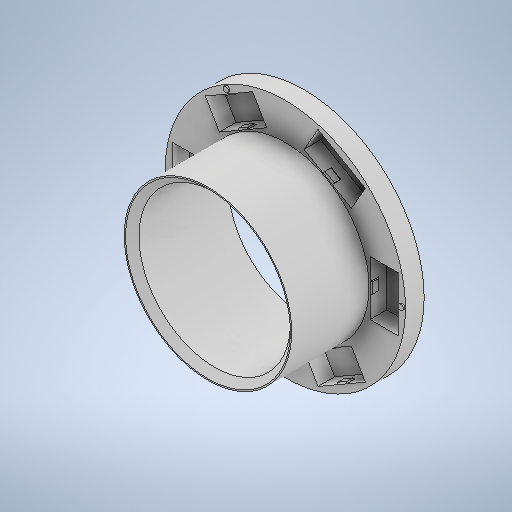
# Autodesk Inventor part: 2.5inchFemale
Saved by Autodesk Inventor 2025.2 (Build 292293000, 293)
## iProperties
Created: 2024-12-23
Part Number: 2.5inchFemale
Material: Generic
Document SubType Name: Modeling
Designer: lidang
Density: 1 g/cm^3
Appearance: Default
Author: lidang
Autodesk Inventor part; units mm, degrees
ref_plane "YZ Plane" through (0, 0, 0) normal (1, 0, 0) x (0, 1, 0)
ref_plane "XZ Plane" through (0, 0, 0) normal (0, 1, 0) x (-1, 0, 0)
ref_plane "XY Plane" through (0, 0, 0) normal (0, 0, 1) x (1, 0, 0)
sketch "Sketch1" plane through (0, 0, 0) normal (0, 0, 1) x (1, 0, 0)
  circle A0 centre (0, 0) radius 28.35
  line L0 (31.75, 10.25) -> (42.25, 10.25)
  line L1 (42.25, 10.25) -> (42.25, -10.25)
  line L2 (42.25, -10.25) -> (31.75, -10.25)
  line L3 (31.75, -10.25) -> (31.75, 10.25)
  circle A1 centre (0, 0) radius 45
  line L4 (42.25, 2) -> (41.75, 2)
  line L5 (41.75, 2) -> (41.75, -2)
  line L6 (41.75, -2) -> (42.25, -2)
  line L7 (42.25, -2) -> (42.25, 2)
  line L8 (37, 10.25) -> (37, -10.25)
  line L9 (31.75, 2) -> (32.25, 2)
  line L10 (32.25, 2) -> (32.25, -2)
  line L11 (32.25, -2) -> (31.75, -2)
  line L12 (31.75, -2) -> (31.75, 2)
  line L13 (19.3929, 37.5896) -> (19.1429, 37.1566)
  line L14 (22.6071, 35.1566) -> (22.8571, 35.5896)
  line L15 (22.8571, 35.5896) -> (19.3929, 37.5896)
  line L16 (19.1429, 37.1566) -> (22.6071, 35.1566)
  line L17 (14.1429, 28.4963) -> (14.3929, 28.9293)
  line L18 (14.3929, 28.9293) -> (17.8571, 26.9293)
  line L19 (17.6071, 26.4963) -> (14.1429, 28.4963)
  line L20 (17.8571, 26.9293) -> (17.6071, 26.4963)
  line L21 (24.7518, 22.3713) -> (6.9982, 32.6213)
  line L22 (30.0018, 31.4646) -> (24.7518, 22.3713)
  line L23 (12.2482, 41.7146) -> (30.0018, 31.4646)
  line L24 (6.9982, 32.6213) -> (12.2482, 41.7146)
  line L25 (-22.8571, 35.5896) -> (-22.6071, 35.1566)
  line L26 (-19.1429, 37.1566) -> (-19.3929, 37.5896)
  line L27 (-19.3929, 37.5896) -> (-22.8571, 35.5896)
  line L28 (-22.6071, 35.1566) -> (-19.1429, 37.1566)
  line L29 (-17.6071, 26.4963) -> (-17.8571, 26.9293)
  line L30 (-17.8571, 26.9293) -> (-14.3929, 28.9293)
  line L31 (-14.1429, 28.4963) -> (-17.6071, 26.4963)
  line L32 (-14.3929, 28.9293) -> (-14.1429, 28.4963)
  line L33 (-6.9982, 32.6213) -> (-24.7518, 22.3713)
  line L34 (-12.2482, 41.7146) -> (-6.9982, 32.6213)
  line L35 (-30.0018, 31.4646) -> (-12.2482, 41.7146)
  line L36 (-24.7518, 22.3713) -> (-30.0018, 31.4646)
  line L37 (-42.25, -2) -> (-41.75, -2)
  line L38 (-41.75, 2) -> (-42.25, 2)
  line L39 (-42.25, 2) -> (-42.25, -2)
  line L40 (-41.75, -2) -> (-41.75, 2)
  line L41 (-31.75, -2) -> (-32.25, -2)
  line L42 (-32.25, -2) -> (-32.25, 2)
  line L43 (-31.75, 2) -> (-31.75, -2)
  line L44 (-32.25, 2) -> (-31.75, 2)
  line L45 (-31.75, 10.25) -> (-31.75, -10.25)
  line L46 (-42.25, 10.25) -> (-31.75, 10.25)
  line L47 (-42.25, -10.25) -> (-42.25, 10.25)
  line L48 (-31.75, -10.25) -> (-42.25, -10.25)
  line L49 (-19.3929, -37.5896) -> (-19.1429, -37.1566)
  line L50 (-22.6071, -35.1566) -> (-22.8571, -35.5896)
  line L51 (-22.8571, -35.5896) -> (-19.3929, -37.5896)
  line L52 (-19.1429, -37.1566) -> (-22.6071, -35.1566)
  line L53 (-14.1429, -28.4963) -> (-14.3929, -28.9293)
  line L54 (-14.3929, -28.9293) -> (-17.8571, -26.9293)
  line L55 (-17.6071, -26.4963) -> (-14.1429, -28.4963)
  line L56 (-17.8571, -26.9293) -> (-17.6071, -26.4963)
  line L57 (-24.7518, -22.3713) -> (-6.9982, -32.6213)
  line L58 (-30.0018, -31.4646) -> (-24.7518, -22.3713)
  line L59 (-12.2482, -41.7146) -> (-30.0018, -31.4646)
  line L60 (-6.9982, -32.6213) -> (-12.2482, -41.7146)
  line L61 (22.8571, -35.5896) -> (22.6071, -35.1566)
  line L62 (19.1429, -37.1566) -> (19.3929, -37.5896)
  line L63 (19.3929, -37.5896) -> (22.8571, -35.5896)
  line L64 (22.6071, -35.1566) -> (19.1429, -37.1566)
  line L65 (17.6071, -26.4963) -> (17.8571, -26.9293)
  line L66 (17.8571, -26.9293) -> (14.3929, -28.9293)
  line L67 (14.1429, -28.4963) -> (17.6071, -26.4963)
  line L68 (14.3929, -28.9293) -> (14.1429, -28.4963)
  line L69 (6.9982, -32.6213) -> (24.7518, -22.3713)
  line L70 (12.2482, -41.7146) -> (6.9982, -32.6213)
  line L71 (30.0018, -31.4646) -> (12.2482, -41.7146)
  line L72 (24.7518, -22.3713) -> (30.0018, -31.4646)
  circle A2 centre (0, 0) radius 31.35
  point P0 (27.3768, 26.9179)
  point P1 (9.6232, 37.1679)
  point P2 (-9.6232, 37.1679)
  point P3 (-27.3768, 26.9179)
  point P4 (-37, 10.25)
  point P5 (-37, -10.25)
  point P6 (-27.3768, -26.9179)
  point P7 (-9.6232, -37.1679)
  point P8 (9.6232, -37.1679)
  point P9 (27.3768, -26.9179)
  dimension "d1" = 56.7
  dimension "d16" = 20.5
  dimension "d17" = 10.5
  dimension "d72" = 10.25
  dimension "d73" = 90
  dimension "d74" = 4
  dimension "d75" = 0.5
  dimension "d76" = 2
  dimension "d83" = 360
  dimension "d85" = 62.7
  dimension "d114" = 37
  constraints: 146 end point, 6 point on line, 4 parallel, 4 symmetric about line, 3 centre point, 2 horizontal, 2 midpoint, 2 perpendicular, 1 coincident, 157 other
  measures "d1" diameter of A0
  measures "d16" distance of L0.end L1.end
  measures "d17" distance of L1.end L2.end
  measures "d72" vertical distance of point (0, 0) L8.start
  measures "d73" diameter of A1
  measures "d74" distance of L4.end L5.end
  measures "d75" distance of L5.end L6.end
  measures "d76" vertical distance of point (0, 0) L5.end
  measures "d85" diameter of A2
  measures "d114" horizontal distance of point (0, 0) L8.start
extrude "Extrusion9" add sketch "Sketch1" along normal blind 7 contours A0 | L0 L8 L2 L3 L11 L10 L9 | L0 L1 L4 L5 L6 L2 L8 | L9 L10 L11 L3 | L1 L6 L5 L4 | A1 | L15 L14 L16 L13 | L13 L16 L14 L23 L22 L21 L20 L18 L17 L24 | L17 L18 L20 L19 | L27 L26 L28 L25 | L25 L28 L26 L35 L34 L33 L32 L30 L29 L36 | L29 L30 L32 L31 | L39 L38 L40 L37 | L37 L40 L38 L47 L46 L45 L44 L42 L41 L48 | L41 L42 L44 L43 | L51 L50 L52 L49 | L49 L52 L50 L59 L58 L57 L56 L54 L53 L60 | L53 L54 L56 L55 | L63 L62 L64 L61 | L61 L64 L62 L71 L70 L69 L68 L66 L65 L72 | L65 L66 L68 L67 | A2
extrude "Extrusion10" add sketch "Sketch1" along normal blind 36 contours A0 | A2
extrude "Extrusion11" cut sketch "Sketch1" along normal blind 36 contours A0
extrude "Extrusion12" cut sketch "Sketch1" along normal blind 7 contours L39 L38 L40 L37 | L37 L40 L38 L47 L46 L45 L44 L42 L41 L48 | L41 L42 L44 L43
extrude "Extrusion13" add sketch "Sketch1" along normal blind 7 contours L39 L38 L40 L37 | L41 L42 L44 L43
extrude "Extrusion14" add sketch "Sketch1" along normal blind 0.75 contours L39 L38 L40 L37 | L37 L40 L38 L47 L46 L45 L44 L42 L41 L48 | L41 L42 L44 L43
chamfer "Chamfer4" distance 0.5 angle 45 1 edges at (-41.75, 0, 7)
pattern_circular "Circular Pattern3" count 6 over 360 about axis through (0, 0, 0) along (0, 0, 1) of "Extrusion12", "Extrusion13", "Extrusion14", "Chamfer4"
chamfer "Chamfer5" distance 2.5 angle 45 1 edges at (-28.35, 0, 36)
sketch "Sketch3" plane through (0, 0, 7) normal (0, 0, 1) x (1, 0, 0)
  circle A0 centre (43.75, 0) radius 1
  line L0 (42.25, -2) -> (42.25, 2) projected
  point P0 (0, 0)
  dimension "d107" = 2
  dimension "d108" = 1.5
  constraints: 1 centre point
  measures "d107" diameter of A0
  measures "d108" distance from line of L0 A0.centre
extrude "Extrusion15" add sketch "Sketch3" along normal blind 0.5
pattern_circular "Circular Pattern4" count 3 over 360 about axis through (0, 0, 0) along (0, 0, 1) of "Extrusion15"
sketch "Sketch4" plane through (0, 0, 0.75) normal (0, 0, 1) x (1, 0, 0)
  line L0 (-41.75, -2) -> (-41.75, 2) projected
  line L1 (-42.25, -2) -> (-41.75, -2) projected
  line L2 (-41.75, 2) -> (-42.25, 2)
  line L3 (-42.25, 2) -> (-42.25, -2)
  line L4 (-42.25, -2) -> (-41.75, -2)
  line L5 (-41.75, -2) -> (-41.75, 2)
  line L6 (-32.25, -2) -> (-31.75, -2) projected
  line L7 (-31.75, -2) -> (-32.25, -2)
  line L8 (-32.25, -2) -> (-32.25, 2)
  line L9 (-32.25, 2) -> (-31.75, 2)
  line L10 (-31.75, 2) -> (-31.75, -2)
  point P0 (0, 0)
  constraints: 16 end point, 4 parallel, 2 horizontal, 2 perpendicular
extrude "Extrusion16" cut sketch "Sketch4" along normal blind 3
pattern_circular "Circular Pattern5" count 6 over 360 about axis through (0, 0, 0) along (0, 0, 1) of "Extrusion16"
chamfer "Chamfer6" distance 0.5 angle 45 18 edges at (-32.25, 0, 3.75) (-20.875, -36.1566, 3.75) (-41.75, 0, 3.75) (-16.125, -27.9293, 3.75) (16.125, -27.9293, 3.75) (20.875, -36.1566, 3.75) (32.25, 0, 3.75) (41.75, 0, 3.75) (20.875, 36.1566, 3.75) (16.125, 27.9293, 3.75) (-16.125, 27.9293, 3.75) (-20.875, 36.1566, 3.75) (-32.25, 0, 7) (-16.125, -27.9293, 7) (16.125, -27.9293, 7) (32.25, 0, 7) (16.125, 27.9293, 7) (-16.125, 27.9293, 7)
equation "\"d72\" = 0.5 * d16"
equation "\"d76\" = 0.5 * d74"
body "Solid2"
